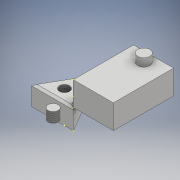
# Autodesk Inventor part: Part2
Saved by Autodesk Inventor 2017 (Build 210142000, 142)
## iProperties
Part Number: Part2
Material: 一般
Document SubType Name: Modeling
Designer: 7989303491
Density: 1 g/cm^3
Appearance: 既定
Author: 7989303491
Autodesk Inventor part; units mm, degrees
ref_plane "YZ Plane" through (0, 0, 0) normal (1, 0, 0) x (0, 1, 0)
ref_plane "XZ Plane" through (0, 0, 0) normal (0, 1, 0) x (-1, 0, 0)
ref_plane "XY Plane" through (0, 0, 0) normal (0, 0, 1) x (1, 0, 0)
sketch "スケッチ2" plane through (0, 0, 0) normal (0, 0, 1) x (1, 0, 0)
  point P0 (0, 0)
sketch "スケッチ3" plane through (0, 0, 0) normal (0, 0, 1) x (1, 0, 0)
  point P0 (0, 0)
sketch "スケッチ4" plane through (0, 0, 0) normal (0, 0, 1) x (1, 0, 0)
  line L0 (-20.7682, 0) -> (0, 0)
  line L1 (0, 0) -> (-10.3841, 17.9858)
  line L2 (-10.3841, 17.9858) -> (-20.7682, 0)
  point P0 (-10.3841, 0)
  constraints: 6 end point, 2 equal length, 1 coincident, 1 horizontal, 1 midpoint
extrude "押し出し1" add sketch "スケッチ4" along normal blind 10
chamfer "面取り1" distance 1 angle 45 1 edges at (-5.1921, 8.9929, 10)
chamfer "面取り2" distance 1 angle 45 2 edges at (-15.8649, 8.4929, 10) (-10.9615, 0, 10)
sketch "スケッチ5" plane through (0, 0, 10) normal (0, 0, 1) x (1, 0, 0)
  line L0 (-10.3841, 15.9858) -> (-10.3841, 17.9858) projected
  circle A0 centre (-10.3841, 5.9953) radius 2.5
  line L1 (-1.7321, 1) -> (-19.0362, 1) projected
  line L2 (-10.3841, 15.9858) -> (-1.7321, 1) projected
  point P0 (0, 0)
  dimension "d9" = 5
  constraints: 2 coincident, 1 centre point, 2 other
  measures "d9" diameter of A0
extrude "押し出し2" cut sketch "スケッチ5" against normal blind 5
chamfer "面取り3" distance 0.2 angle 45 1 edges at (-12.8841, 5.9953, 5)
thread "ねじ1" size "M5x0.8" class "6H" standard "ANSI Metric M Profile" full length
sketch "スケッチ6" plane through (0, 0, 10) normal (0, 0, 1) x (1, 0, 0)
  circle A0 centre (0, -10.0364) radius 2.5
  point P0 (0, 0)
  dimension "d17" = 5
  constraints: 1 centre point
  measures "d17" diameter of A0
extrude "押し出し3" add sketch "スケッチ6" along normal blind 5
thread "ねじ2" size "M5x0.8" class "6g" standard "ANSI Metric M Profile" full length
sketch "スケッチ7" plane through (0, -10.0364, 15) normal (0, 0, 1) x (1, 0, 0)
  point P0 (0, 10.0364)
sketch "スケッチ8" plane through (0, 0, 10) normal (0, 0, 1) x (1, 0, 0)
  point P0 (0, 0)
sketch "スケッチ9" plane through (-20.7682, 0, 9) normal (0, -0.7071, 0.7071) x (1, 0, 0)
  point P0 (20.7682, -6.364)
sketch "スケッチ10" plane through (-20.7682, 0, 0) normal (0, -1, 0) x (1, 0, 0)
  point P0 (20.7682, 0)
sketch "スケッチ11" plane through (0, 0, 10) normal (0, 0, 1) x (1, 0, 0)
  line L0 (0, 0) -> (-1.7321, 1) projected
  line L1 (0, 0) -> (19.954, 0)
  line L2 (19.954, 0) -> (19.954, 29.9824)
  line L3 (19.954, 29.9824) -> (0, 29.9824)
  line L4 (0, 29.9824) -> (0, 0)
  constraints: 8 end point, 1 horizontal, 1 parallel
extrude "押し出し4" add sketch "スケッチ11" along normal blind 12
sketch "スケッチ12" plane through (0, 0, 22) normal (0, 0, 1) x (1, 0, 0)
  point P0 (0, 0)
sketch "スケッチ13" plane through (0, 0, 22) normal (0, 0, 1) x (1, 0, 0)
  circle A0 centre (10.0005, 25.13) radius 3
  point P0 (0, 0)
  dimension "d24" = 6
  constraints: 1 centre point
  measures "d24" diameter of A0
extrude "押し出し5" add sketch "スケッチ13" along normal blind 4
sketch "スケッチ14" plane through (0, 0, 22) normal (0, 0, 1) x (1, 0, 0)
  point P0 (0, 0)
